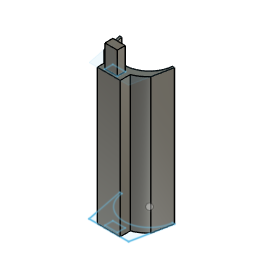
STEAM Rollercoasters Rail v2 (Autodesk Fusion 360 design; units mm, degrees)
Autodesk Fusion 360 part; units mm, degrees
sketch "Sketch1" plane through (0, 0, 0) normal (0, 0, 1) x (1, 0, 0)
  line L0 (17.5, -25) -> (-17.5, -25)
  line L1 (5.5, -23) -> (-5.5, -23)
  line L2 (-5.5, -23) -> (-5.5, -16)
  line L3 (-5.5, -16) -> (5.5, -16)
  line L4 (5.5, -16) -> (5.5, -23)
  line L5 (-24.2785, 8.8924) -> (-22.4011, 8.8924)
  line L6 (-17.5, -25) -> (-24.2785, 8.8924)
  line L7 (22.4011, 8.8924) -> (24.2781, 8.8924)
  line L8 (24.2781, 8.8924) -> (17.5, -25)
  arc A0 (-22.4011, 8.8924) -> (22.4011, 8.8924) centre (0, 11) ccw
  dimension "d4" = 45
  dimension "d5" = 1.877
  constraint horizontal L1
  constraint vertical L2
  constraint horizontal L3
  constraint vertical L4
  constraint horizontal L5
  constraint parallel L5 L7
  measures "d4" diameter of A0
  measures "d5" distance of L7.start L7.end
extrude "Extrude1" add sketch "Sketch1" along normal blind 120
extrude "Extrude2" add sketch "Sketch1" along normal blind 120 contours L1 L2 L3 L4
extrude "Extrude3" cut sketch "Sketch1" along normal blind 20 contours L1 L2 L3 L4
sketch "Sketch2" plane through (0, 0, 120) normal (0, 0, 1) x (-1, 0, 0)
  line L0 (22.4011, -8.8924) -> (24.2785, -8.8924)
  line L1 (24.2785, -8.8924) -> (17.5, 25)
  line L2 (17.5, 25) -> (-17.5, 25)
  line L3 (-17.5, 25) -> (-24.2781, -8.8924)
  line L4 (-24.2781, -8.8924) -> (-22.4011, -8.8924)
  arc A0 (22.4011, -8.8924) -> (-22.4011, -8.8924) centre (0, -11) ccw
  line L5 (-5.5, 23) -> (5.5, 23)
  line L6 (5.5, 23) -> (5.5, 16)
  line L7 (5.5, 16) -> (-5.5, 16)
  line L8 (-5.5, 16) -> (-5.5, 23)
  constraint horizontal L5
  constraint vertical L6
  constraint horizontal L7
  constraint vertical L8
extrude "Extrude4" add sketch "Sketch2" along normal blind 20 contours L5 L6 L7 L8
sketch "Sketch3" plane through (0, 0, 0) normal (0, 0, 1) x (1, 0, 0)
  circle A0 centre (0, 10) radius 27.8887
  line L0 (-10.2931, -15.9198) -> (-10.2931, -26.4867)
  line L1 (-10.2931, -26.4867) -> (10, -26.4867)
  line L2 (10, -26.4867) -> (10, -16.0342)
  line L3 (-10.2931, -26.4867) -> (-25, -26.4867)
  line L4 (-25, -26.4867) -> (-25, -2.3605)
  line L5 (10, -26.4867) -> (25, -26.4867)
  line L6 (25, -26.4867) -> (25, -2.3605)
  constraint coincident A0 L0.start
  constraint vertical L0
  constraint perpendicular L0 L1
  constraint coincident A0 L2.end
  constraint perpendicular L1 L2
  constraint perpendicular L0 L3
  constraint coincident A0 L4.end
  constraint perpendicular L1 L4
  constraint perpendicular L2 L5
  constraint coincident A0 L6.end
  constraint perpendicular L5 L6
extrude "Extrude5" cut sketch "Sketch3" along normal blind 135 contours A0 L0 L3 L4 | A0 L2 L5 L6
